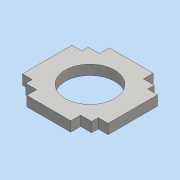
# Autodesk Inventor part: Camera-Holder_Bearing-Ring-Middle
Saved by Autodesk Inventor 2016 SP1 (Build 200210100, 210)
## iProperties
Created: 2016-01-20
Part Number: Camera-Holder_Bearing-Ring-Middle
Material: Generic
Document SubType Name: Modeling
Designer: Mohamed A.
Density: 1 g/cm^3
Appearance: Default
Author: Mohamed A.
Autodesk Inventor part; units mm, degrees
ref_plane "YZ Plane" through (0, 0, 0) normal (1, 0, 0) x (0, 1, 0)
ref_plane "XZ Plane" through (0, 0, 0) normal (0, 1, 0) x (-1, 0, 0)
ref_plane "XY Plane" through (0, 0, 0) normal (0, 0, 1) x (1, 0, 0)
sketch "Sketch1" plane through (0, 0, 0) normal (0, 0, 1) x (1, 0, 0)
  circle A0 centre (0, 0) radius 7.5
  line L0 (12.9997, 7.5) -> (9.9997, 7.5)
  line L1 (9.9997, 7.5) -> (9.9997, 9.5)
  line L2 (9.9997, -9.5) -> (9.9997, -7.5)
  line L3 (9.9997, -7.5) -> (12.9997, -7.5)
  line L4 (-6.667, -12.5) -> (-6.667, -9.5)
  line L5 (-6.667, -9.5) -> (-10.0003, -9.5)
  line L6 (6.6663, -12.5) -> (6.6663, -9.5)
  line L7 (6.6663, -9.5) -> (9.9997, -9.5)
  line L8 (-13.0003, -7.5) -> (-10.0003, -7.5)
  line L9 (-10.0003, -7.5) -> (-10.0003, -9.5)
  line L10 (-13.0003, 7.5) -> (-10.0003, 7.5)
  line L11 (-10.0003, 7.5) -> (-10.0003, 9.5)
  line L12 (-6.667, 12.5) -> (-6.667, 9.5)
  line L13 (-6.667, 9.5) -> (-10.0003, 9.5)
  line L14 (9.9997, 9.5) -> (6.6663, 9.5)
  line L15 (6.6663, 9.5) -> (6.6663, 12.5)
  line L16 (12.9997, 7.5) -> (12.9997, -7.5)
  line L17 (-6.667, 12.5) -> (6.6663, 12.5)
  line L18 (-13.0003, -7.5) -> (-13.0003, 7.5)
  line L19 (6.6663, -12.5) -> (-6.667, -12.5)
  line L20 (12.9997, -7.5) -> (12.9997, 7.5)
  line L21 (-20.9424, 0) -> (31.3224, 0) construction
  line L22 (-0.0003, 36) -> (-0.0003, -23) construction
  dimension "d0" = 15
  dimension "d3" = 3
  dimension "d5" = 3
  dimension "d6" = 3
  dimension "d15" = 25
  dimension "d16" = 3
  dimension "d18" = 20
  dimension "d19" = 13.3333
  dimension "d20" = 15
  constraints: 46 end point, 12 point on line, 8 perpendicular, 4 horizontal, 3 collinear, 2 parallel, 2 vertical, 1 centre point, 1 coincident, 2 other
  measures "d0" diameter of A0
  measures "d3" distance of L0.start L0.end
  measures "d5" distance of L8.start L8.end
  measures "d6" distance of L12.start L12.end
  measures "d15" distance between parallel lines of L19 L17
  measures "d16" distance of L6.start L6.end
  measures "d18" distance between parallel lines of L11 L1
  measures "d19" distance between parallel lines of L12 L15
  measures "d20" distance of L20.start L0.start
extrude "Extrusion1" add sketch "Sketch1" along normal mid plane 3
equation "\"d19\" = 0.666667 * d18"
body "Solid1"
